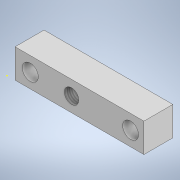
# Autodesk Inventor part: block
Saved by Autodesk Inventor 2021 (Build 250183000, 183)
## iProperties
Created: 2021-02-05
Part Number: block
Material: Generic
Document SubType Name: Modeling
Designer: nevkd
Density: 1 g/cm^3
Appearance: Default
Author: nevkd
Autodesk Inventor part; units mm, degrees
ref_plane "YZ Plane" through (0, 0, 0) normal (1, 0, 0) x (0, 1, 0)
ref_plane "XZ Plane" through (0, 0, 0) normal (0, 1, 0) x (-1, 0, 0)
ref_plane "XY Plane" through (0, 0, 0) normal (0, 0, 1) x (1, 0, 0)
sketch "Sketch1" plane through (0, 0, 0) normal (0, 0, 1) x (1, 0, 0)
  line L0 (0, 0) -> (100, 0)
  line L1 (100, 0) -> (100, 20)
  line L2 (100, 20) -> (0, 20)
  line L3 (0, 20) -> (0, 0)
  dimension "d0" = 100
  dimension "d1" = 20
  constraints: 8 end point, 2 parallel, 1 horizontal, 1 perpendicular
  measures "d0" distance of L0.start L0.end
  measures "d1" distance of L2.end L0.start
extrude "Extrusion1" add sketch "Sketch1" against normal blind 20
sketch "Sketch2" plane through (0, 0, 0) normal (0, 0, 1) x (1, 0, 0)
  line L0 (0, 0) -> (0, 20) projected
  circle A0 centre (44.5, 10) radius 5
  line L1 (0, 0) -> (100, 0) projected
  dimension "d5" = 10
  dimension "d24" = 44.5
  dimension "d25" = 10
  constraints: 1 centre point
  measures "d5" diameter of A0
  measures "d24" distance from line of L0 A0.centre
  measures "d25" distance from line of L1 A0.centre
sketch "Sketch3" plane through (0, 0, 0) normal (0, 0, 1) x (1, 0, 0)
  line L0 (0, 0) -> (0, 20) projected
  line L1 (100, 20) -> (100, 0) projected
  line L2 (100, 10) -> (85.3, 10)
  circle A0 centre (85.3, 10) radius 5.5
  dimension "d8" = 14.7
  dimension "d9" = 11
  constraints: 2 end point, 1 centre point, 1 coincident, 1 horizontal, 1 midpoint
  measures "d8" distance of L2.start L2.end
  measures "d9" diameter of A0
extrude "Extrusion2" cut sketch "Sketch3" against normal blind 20
extrude "Extrusion3" cut sketch "Sketch2" against normal blind 20
sketch "Sketch4" plane through (0, 0, 0) normal (0, 0, 1) x (1, 0, 0)
  line L0 (0, 20) -> (0, 0) projected
  circle A0 centre (16, 10) radius 5.5
  circle A1 centre (44.5, 10) radius 5 projected
  line L1 (0, 0) -> (100, 0) projected
  dimension "d15" = 11
  dimension "d27" = 10
  dimension "d29" = 16
  constraints: 1 centre point
  measures "d15" diameter of A0
  measures "d27" distance from line of L1 A0.centre
  measures "d29" distance from line of A0.centre L0
extrude "Extrusion4" cut sketch "Sketch4" against normal blind 20 contours A0
sketch "Sketch5" plane through (0, 0, 0) normal (0, 0, 1) x (1, 0, 0)
  point P0 (0, 0)
sketch "Sketch6" plane through (100, 0, 0) normal (1, 0, 0) x (0, 0, -1)
  line L0 (0, 0) -> (20, 0) projected
  line L1 (20, 0) -> (20, 20) projected
  line L2 (0, 0) -> (20, 0)
  line L3 (20, 0) -> (20, 20)
  line L4 (20, 20) -> (0, 20)
  line L5 (0, 20) -> (0, 0)
  constraints: 8 end point, 2 parallel, 1 horizontal, 1 perpendicular
extrude "Extrusion5" cut sketch "Sketch6" against normal blind 5.5
sketch "Sketch7" plane through (0, 0, 0) normal (-1, 0, 0) x (0, 0, 1)
  line L0 (-20, 0) -> (-20, 20) projected
  line L1 (0, 20) -> (-20, 20) projected
  line L2 (-20, 0) -> (0, 0)
  line L3 (0, 0) -> (0, 20)
  line L4 (0, 20) -> (-20, 20)
  line L5 (-20, 20) -> (-20, 0)
  constraints: 8 end point, 2 parallel, 1 horizontal, 1 perpendicular
extrude "Extrusion6" cut sketch "Sketch7" against normal blind 5.5
thread "Thread1" size "M10x1.5" class "6H" standard "ANSI Metric M Profile" full length
body "Solid1"
